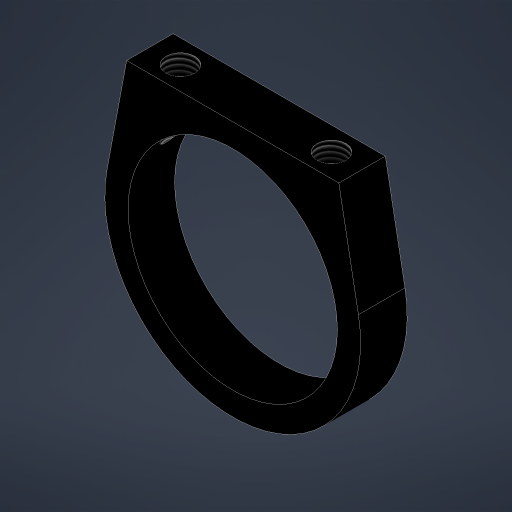
# Autodesk Inventor part: Tarot_12mm_Mount
Saved by Autodesk Inventor 2024 (Build 280153000, 153)
## iProperties
Created: 2023-06-28
Part Number: Tarot_12mm_Mount
Material: Aluminum 6061
Document SubType Name: Modeling
Designer: dzw04
Density: 2.7 g/cm^3
Appearance: Anodized - Black
Author: dzw04
Autodesk Inventor part; units mm, degrees
ref_plane "YZ Plane" through (0, 0, 0) normal (1, 0, 0) x (0, 1, 0)
ref_plane "XZ Plane" through (0, 0, 0) normal (0, 1, 0) x (-1, 0, 0)
ref_plane "XY Plane" through (0, 0, 0) normal (0, 0, 1) x (1, 0, 0)
sketch "Sketch1" plane through (0, 0, 0) normal (0, 0, 1) x (1, 0, 0)
  circle A0 centre (0, 0) radius 9
  circle A1 centre (0, 0) radius 11
  line L0 (-9.125, 11) -> (9.125, 11)
  line L1 (0, 0) -> (0, 11) construction
  line L2 (-9.125, 11) -> (-10.8107, 2.0321)
  line L3 (9.125, 11) -> (10.8107, 2.0321)
  dimension "d0" = 18
  dimension "d1" = 22
  dimension "d2" = 18.25
  constraints: 8 end point, 3 point on circle, 2 centre point, 2 coincident, 2 tangent, 1 horizontal, 1 midpoint, 1 vertical
  measures "d0" diameter of A0
  measures "d1" diameter of A1
  measures "d2" distance of L0.start L0.end
extrude "Extrusion1" add sketch "Sketch1" along normal blind 4
sketch "Sketch2" plane through (-9.125, 11, 0) normal (0, 1, 0) x (1, 0, 0)
  line L0 (18.25, -4) -> (0, -4) construction
  line L1 (9.125, -4) -> (9.125, 0) construction
  line L2 (9.125, -2) -> (2.625, -2) construction
  line L3 (2.625, -2) -> (15.625, -2) construction
  circle A0 centre (2.625, -2) radius 1.25
  circle A1 centre (15.625, -2) radius 1.25
  dimension "d5" = 6.5
  dimension "d6" = 13
  dimension "d7" = 2.5
  dimension "d8" = 2.5
  constraints: 6 end point, 2 centre point, 2 coincident, 2 midpoint, 1 horizontal, 1 point on line, 1 vertical
  measures "d5" distance of L2.start L2.end
  measures "d6" distance of L2.end L3.end
  measures "d7" diameter of A0
  measures "d8" diameter of A1
extrude "Extrusion2" cut sketch "Sketch2" against normal blind 11
thread "Thread1" size "M2.5x0.45" class "6H" standard "ANSI Metric M Profile" full length
thread "Thread2" size "M2.5x0.45" class "6H" standard "ANSI Metric M Profile" full length
equation "\"d6\" = 2 * d5"
body "Solid1"
